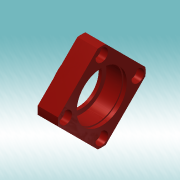
# Autodesk Inventor part: BGSRB6201ZZ_h
Saved by Autodesk Inventor 2015 (Build 190159000, 159)
## iProperties
Category: PARTsolutions
Company: MISUMI
Created: 2016-03-21
Part Number: BGSRB6201ZZ_h
Catalog Web Link: www.cadenas.de
Description: BGSRB, BGSR, BASR, SBASR, SBGSR_housing-Bearings with Housings - Pilot, Retained - Square
Vendor: MISUMI
Document SubType Name: Modeling
Designer: psAdmin
Manufacturer: MISUMI
Mass: 13.0051 g
Surface Area: 73.4993 cm^2
Volume: 13.0051 cm^3
Density: 1 g/cm^3
Material: 一般
Appearance: オレンジ-赤
PSOL_IDENT_0: {$CADENAS_DATA\23d-libs\misumi\metric\12_bearing_holders\bgsrb\bgsrb_housing.prj},223 {VTYP=3D},{NB=
PSOL_IDENT_1: BGSRB6201ZZ_h},{LINA=BGSRB6201ZZ},{NN=BGSRB, BGSR, BASR, SBASR, SBGSR_housing},{DATE=06.11.2015 04:4
PSOL_IDENT_2: 5:35},{GEOMDATE=02.11.2015 07:20:17},{VERSION=},{LINEID=170},{LINESUBID=-1},{WBVAR=MATB,MATH,STH,SEA
PSOL_IDENT_3: L,ALT1}  {NB=BGSRB6201ZZ_h},{LINA=BGSRB6201ZZ},{KT=DUMMY},{PN=BGSRB6201ZZ},{TYPE=BGSRB},{MATB=S},{MA
PSOL_IDENT_4: TBALG= 'S' , 'Steel' , 'SS', 'Stainless Steel' },{MATH=S45C},{MATHALG= 'S45C' , 'S45C' , 'A2017' , '
PSOL_IDENT_5: A2017' },{STH=BO},{STHALG= 'BO','Black Oxide' , 'ENP','Electroless Nickel Plating' },{ARR=Spring Ste
PSOL_IDENT_6: el},{ARRASM=},{BN=6201},{SEAL=ZZ},{SEALALG= 'ZZ','Double Shielded','VV','Non-Contact Sealed Rubber S
PSOL_IDENT_7: eal','DD','Contact Sealed Rubber Seal' },{DD=12},{D=32},{B=10},{H=56},{T=15},{T1=13},{S=2},{LL1=2},{
PSOL_IDENT_8: DDHH=26},{D1=38},{PCD=46},{K=43},{M=M5(4.3)},{DD1=8.0},{H1=4.4},{M3D=5},{BDD2=33.7},{MM=1.35},{ALT1=
PSOL_IDENT_9: }
NN: BGSRB, BGSR, BASR, SBASR, SBGSR_housing
NT: Bearings with Housings - Pilot, Retained - Square
NB: BGSRB6201ZZ_h
NBSYN: $PN._h
LINA: BGSRB6201ZZ
PN: BGSRB6201ZZ
MATB: Steel
MATH: S45C
STH: Black Oxide
ARR: Spring Steel
BN: 6201
SEAL: Double Shielded
DD: 12
D: 32
B: 10
H: 56
T: 15
T1: 13
S: 2
LL1: 2
DDHH: 26
D1: 38
PCD: 46
K: 43
M: M5(4.3)
DD1: 8.0
H1: 4.4
ALT1: Bearing and Retaining Ring Assembled
SUPPLIER: MISUMI
ARTICLENO: BGSRB6201ZZ_h
BOMINFO: BGSRB6201ZZ
CREATOR: CADENAS GmbH
Title: BGSRB6201ZZ
Author: Cadenas PARTsolutions
Comments: Bearings with Housings - Pilot, Retained - Square
Autodesk Inventor part; units mm, degrees
ref_plane "YZ Plane" through (0, 0, 0) normal (1, 0, 0) x (0, 1, 0)
ref_plane "XZ Plane" through (0, 0, 0) normal (0, 1, 0) x (-1, 0, 0)
ref_plane "XY Plane" through (0, 0, 0) normal (0, 0, 1) x (1, 0, 0)
sketch "Sketch_7" plane through (0, 0, 0) normal (0, 0, 1) x (1, 0, 0)
  line L0 (7.5, 0) -> (-7.5, 0)
  line L1 (-7.5, 0) -> (-7.5, 19)
  line L2 (-7.5, 19) -> (-5.8, 19)
  arc A0 (-5.8, 19) -> (-5.5, 19.3) centre (-5.8, 19.3) ccw
  line L3 (-5.5, 19.3) -> (-5.5, 28)
  line L4 (-5.5, 28) -> (7.5, 28)
  line L5 (7.5, 28) -> (7.5, 0)
  line L6 (7.5, 0) -> (-7.5, 0)
  constraints: 14 end point, 2 point on circle, 1 centre point
revolve "Revolution1" add sketch "Sketch_7" angle 360 about axis through (7.5, 0, 0) along (1, 0, 0)
sketch "Sketch_1" plane through (0, 0, 0) normal (0, 0, 1) x (1, 0, 0)
  line L0 (7.5, 0) -> (-7.5, 0)
  line L1 (-7.5, 0) -> (-7.5, 13)
  line L2 (-7.5, 13) -> (-5.5, 13)
  line L3 (-5.5, 13) -> (-5.5, 16)
  line L4 (-5.5, 16) -> (4.5, 16)
  line L5 (4.5, 16) -> (4.5, 16.85)
  line L6 (4.5, 16.85) -> (5.85, 16.85)
  line L7 (5.85, 16.85) -> (5.85, 16)
  line L8 (5.85, 16) -> (7.5, 16)
  line L9 (7.5, 16) -> (7.5, 0)
  line L10 (7.5, 0) -> (-7.5, 0)
  constraints: 22 end point
revolve "Revolution2" cut sketch "Sketch_1" angle 360 about axis through (7.5, 0, 0) along (1, 0, 0)
sketch "Sketch_2" plane through (0, 0, 0) normal (0, 0, 1) x (1, 0, 0)
  line L0 (7.5, 23) -> (-5.5, 23)
  line L1 (-5.5, 23) -> (-5.5, 25.5)
  line L2 (-5.5, 25.5) -> (-5.067, 25.067)
  line L3 (-5.067, 25.067) -> (2.667, 25.067)
  line L4 (2.667, 25.067) -> (3.1, 25.5)
  line L5 (3.1, 25.5) -> (3.1, 27)
  line L6 (3.1, 27) -> (7.5, 27)
  line L7 (7.5, 27) -> (7.5, 23)
  line L8 (7.5, 23) -> (-5.5, 23)
  constraints: 18 end point
revolve "Revolution3" cut sketch "Sketch_2" angle 360 about axis through (7.5, 23, 0) along (1, 0, 0)
thread "Thread1" size "M5x0.8" class "6H" standard "ISO Metric profile" full length
sketch "Sketch_4" plane through (7.5, 0, 0) normal (1, 0, 0) x (0, 0, -1)
  circle A0 centre (0, 0) radius 118.9529
  line L0 (-30.4056, 0) -> (0, -30.4056)
  line L1 (0, -30.4056) -> (30.4056, 0)
  line L2 (30.4056, 0) -> (0, 30.4056)
  line L3 (0, 30.4056) -> (-30.4056, 0)
  constraints: 8 end point, 1 centre point
extrude "Extrusion1" cut sketch "Sketch_4" against normal blind 15
pattern_linear "Rectangular Pattern1" count 2 spacing 32.5269 along (0, -0.7071068, 0.7071068) count 2 spacing 32.5269 along (0, -0.7071068, -0.7071068) of "Revolution3"
ref_plane "housing_to_dummy_XY" through (-7.5, 0, 0) normal (0, 0, 1) x (1, 0, 0)
ref_plane "housing_to_dummy_YZ" through (-7.5, 0, 0) normal (1, 0, 0) x (0, 1, 0)
ref_plane "housing_to_dummy_ZX" through (-7.5, 0, 0) normal (0, 1, 0) x (0, 0, 1)
ref_plane "to_bearings_XY" through (-5.5, 0, 0) normal (-1, 0, 0) x (0, 0, -1)
ref_plane "to_bearings_YZ" through (-5.5, 0, 0) normal (0, 0, -1) x (0, -1, 0)
ref_plane "to_bearings_ZX" through (-5.5, 0, 0) normal (0, -1, 0) x (-1, 0, 0)
ref_plane "to_rring_XY" through (4.5, 0, 0) normal (-1, 0, 0) x (0, 0, -1)
ref_plane "to_rring_YZ" through (4.5, 0, 0) normal (0, 0, -1) x (0, -1, 0)
ref_plane "to_rring_ZX" through (4.5, 0, 0) normal (0, -1, 0) x (-1, 0, 0)
body "Solid1"
